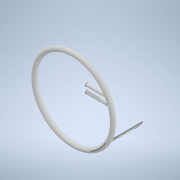
# Autodesk Inventor part: DewarObstructions
Saved by Autodesk Inventor 2020 (Build 240168000, 168)
## iProperties
Created: 2020-09-25
Part Number: DewarObstructions
Material: Generic
Document SubType Name: Modeling
Designer: Eric
Density: 1 g/cm^3
Appearance: Default
Author: Eric
Autodesk Inventor part; units mm, degrees
sketch "Sketch1" plane through (0, 0, 0) normal (1, 0, 0) x (0, 1, 0)
  circle A0 centre (215.9, 69.85) radius 12.7
  line L0 (0, -16.51) -> (0, 99.06) projected
  point P0 (0, 0)
  dimension "d0" = 25.4
  dimension "d1" = 215.9
  dimension "d2" = 69.85
  constraints: 1 centre point
  measures "d0" diameter of A0
  measures "d1" horizontal distance of point (0, 0) A0.centre
  measures "d2" vertical distance of point (0, 0) A0.centre
revolve "Revolution1" add sketch "Sketch1" angle 360 about axis through (0, 0, -10) along (0, 0, 1)
ref_plane "Work Plane1" through (114.3, 0, 0) normal (1, 0, 0) x (0, 1, 0)
sketch "Sketch2" plane through (114.3, 0, 0) normal (1, 0, 0) x (0, 1, 0)
  circle A0 centre (0, 0) radius 7.5
  line L0 (-320.04, 0) -> (320.04, 0) projected
  circle A1 centre (35, 0) radius 7.5
  dimension "d5" = 15
  dimension "d6" = 15
  dimension "d7" = 35
  constraints: 2 centre point, 1 coincident, 1 point on line
  measures "d5" diameter of A0
  measures "d6" diameter of A1
  measures "d7" distance of A0.centre A1.centre
extrude "Extrusion1" add sketch "Sketch2" against normal up to surface (114.3 mm away)
ref_plane "Work Plane2" through (0, -100, 0) normal (0, 1, 0) x (-1, 0, 0)
ref_plane "Work Plane3" through (0, 0, 0) normal (0.5, 0.866, 0) x (0, 0, 1)
sketch "Sketch4" plane through (0, 0, 0) normal (0.5, 0.866, 0) x (0, 0, 1)
  line L0 (82.55, 215.9) -> (82.55, -215.9) projected
  line L1 (-120.65, 216.9) -> (82.55, 216.9)
  line L2 (82.55, 216.9) -> (82.55, 214.9)
  line L3 (82.55, 214.9) -> (-120.65, 214.9)
  line L4 (-120.65, 214.9) -> (-120.65, 216.9)
  line L5 (-161.29, 0) -> (123.19, 0) projected
  point P0 (0, 0)
  dimension "d15" = 2
  dimension "d16" = 203.2
  constraints: 8 end point, 2 parallel, 1 horizontal, 1 midpoint, 1 perpendicular
  measures "d15" distance of L3.end L1.start
  measures "d16" distance of L1.start L1.end
revolve "Revolution3" add sketch "Sketch4" angle 30 about axis through (0, 0, -10) along (0, 0, -1)
body "Solid1"
